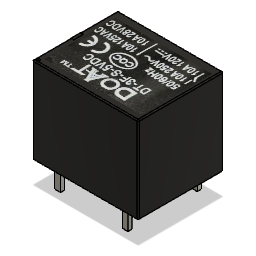
DOAT 5VOLT RELAY v1 (Autodesk Fusion 360 design; units mm, degrees)
Autodesk Fusion 360 part; units mm, degrees
sketch "Sketch1" plane through (0, 0, 0) normal (0, 1, 0) x (1, 0, 0)
  line L0 (9.375, -7.575) -> (-9.375, -7.575)
  line L1 (-9.375, -7.575) -> (-9.375, 7.575)
  line L2 (-9.375, 7.575) -> (9.375, 7.575)
  line L3 (9.375, 7.575) -> (9.375, -7.575)
  line L4 (9.375, -7.575) -> (-9.375, 7.575) construction
  line L5 (-9.375, -7.575) -> (9.375, 7.575) construction
  dimension "d1" = 15.15
  dimension "d2" = 18.75
  constraint horizontal L0
  constraint perpendicular L0 L1
  constraint parallel L0 L2
  constraint parallel L1 L3
  constraint coincident L4 origin
  constraint coincident L5 origin
  measures "d1" distance of L0.end L1.end
  measures "d2" distance of L1.end L2.end
extrude "Extrude1" add sketch "Sketch1" along normal blind 15.24
fillet "Fillet1" radius 0.2 4 edges at (9.375, 7.62, 7.575) (-9.375, 7.62, 7.575) (-9.375, 7.62, -7.575) (9.375, 7.62, -7.575) 1 faces at (3.125, 15.24, 2.525)
sketch "Sketch2" plane through (0, 0, 0) normal (0, -1, 0) x (1, 0, 0)
  arc A0 (-9.375, -7.375) -> (-9.175, -7.575) centre (-9.175, -7.375) ccw
  line L0 (-9.175, -7.575) -> (9.175, -7.575)
  arc A1 (9.175, -7.575) -> (9.375, -7.375) centre (9.175, -7.375) ccw
  line L1 (9.375, -7.375) -> (9.375, 7.375)
  arc A2 (9.375, 7.375) -> (9.175, 7.575) centre (9.175, 7.375) ccw
  line L2 (9.175, 7.575) -> (-9.175, 7.575)
  arc A3 (-9.175, 7.575) -> (-9.375, 7.375) centre (-9.175, 7.375) ccw
  line L3 (-9.375, 7.375) -> (-9.375, -7.375)
  line L4 (6.5, -6.5) -> (-6.5, -6.5) construction
  line L5 (-6.5, -6.5) -> (-6.5, 6.5) construction
  line L6 (-6.5, 6.5) -> (6.5, 6.5) construction
  line L7 (6.5, 6.5) -> (6.5, -6.5) construction
  line L8 (6.5, -6.5) -> (-6.5, 6.5) construction
  line L9 (-6.5, -6.5) -> (6.5, 6.5) construction
  line L10 (-6.5, 6.5) -> (-5.5, 6.5)
  line L11 (-5.5, 6.5) -> (-5.5, 5.8)
  line L12 (-5.5, 5.8) -> (-6.5, 5.8)
  line L13 (-6.5, 5.8) -> (-6.5, 6.5)
  line L14 (6.5, 5.8) -> (5.5, 5.8)
  line L15 (5.5, 6.5) -> (6.5, 6.5)
  line L16 (5.5, 5.8) -> (5.5, 6.5)
  line L17 (6.5, 6.5) -> (6.5, 5.8)
  line L18 (-5.5, -6.5) -> (-6.5, -6.5)
  line L19 (-6.5, -5.8) -> (-5.5, -5.8)
  line L20 (-6.5, -6.5) -> (-6.5, -5.8)
  line L21 (-5.5, -5.8) -> (-5.5, -6.5)
  line L22 (6.5, -6.5) -> (5.5, -6.5)
  line L23 (5.5, -5.8) -> (6.5, -5.8)
  line L24 (5.5, -6.5) -> (5.5, -5.8)
  line L25 (6.5, -5.8) -> (6.5, -6.5)
  dimension "d7" = 13
  dimension "d8" = 13
  dimension "d9" = 1
  dimension "d10" = 0.7
  dimension "d13" = 12
  dimension "d14" = -12.3
  constraint horizontal L4
  constraint perpendicular L4 L5
  constraint parallel L4 L6
  constraint parallel L5 L7
  constraint coincident L8 origin
  constraint coincident L9 origin
  constraint horizontal L10
  constraint vertical L11
  constraint horizontal L12
  constraint vertical L13
  measures "d7" distance of L5.end L6.end
  measures "d8" distance of L4.end L5.end
  measures "d9" distance of L5.end L10.end
  measures "d10" distance of L5.end L12.end
extrude "Extrude2" add sketch "Sketch2" along normal blind 4 contours L10 L11 L12 L13 | L14 L15 L16 L17 | L18 L19 L20 L21 | L22 L23 L24 L25
chamfer "Chamfer1" distance 0.2 angle 45 8 edges at (5.5, -4, 6.15) (6, -4, 6.5) (6.5, -4, 6.15) (6, -4, 5.8) (6, -4, -5.8) (6.5, -4, -6.15) (6, -4, -6.5) (5.5, -4, -6.15) 2 faces at (-6.1667, -4, 6.2667) (-5.8333, -4, -6.2667)
sketch "Sketch3" plane through (0, 0, 0) normal (0, -1, 0) x (1, 0, 0)
  line L0 (6.5, -5.8) -> (6.5, -6.5)
  line L1 (6.5, -6.5) -> (5.5, -6.5)
  line L2 (5.5, -6.5) -> (5.5, -5.8)
  line L3 (5.5, -5.8) -> (6.5, -5.8)
  line L4 (-6.5, 5.8) -> (-6.5, 6.5)
  line L5 (-6.5, 6.5) -> (-5.5, 6.5)
  line L6 (-5.5, 6.5) -> (-5.5, 5.8)
  line L7 (-5.5, 5.8) -> (-6.5, 5.8)
  line L8 (-5.5, -5.8) -> (-5.5, -6.5)
  line L9 (-5.5, -6.5) -> (-6.5, -6.5)
  line L10 (-6.5, -6.5) -> (-6.5, -5.8)
  line L11 (-6.5, -5.8) -> (-5.5, -5.8)
  line L12 (6.5, 6.5) -> (6.5, 5.8)
  line L13 (6.5, 5.8) -> (5.5, 5.8)
  line L14 (5.5, 5.8) -> (5.5, 6.5)
  line L15 (5.5, 6.5) -> (6.5, 6.5)
  arc A0 (-9.375, -7.375) -> (-9.175, -7.575) centre (-9.175, -7.375) ccw
  line L16 (-9.175, -7.575) -> (9.175, -7.575)
  arc A1 (9.175, -7.575) -> (9.375, -7.375) centre (9.175, -7.375) ccw
  line L17 (9.375, -7.375) -> (9.375, 7.375)
  arc A2 (9.375, 7.375) -> (9.175, 7.575) centre (9.175, 7.375) ccw
  line L18 (9.175, 7.575) -> (-9.175, 7.575)
  arc A3 (-9.175, 7.575) -> (-9.375, 7.375) centre (-9.175, 7.375) ccw
  line L19 (-9.375, 7.375) -> (-9.375, -7.375)
  line L20 (0, 0) -> (-9.375, 0) construction
  line L21 (-7.375, -0.5) -> (-8.075, -0.5)
  line L22 (-8.075, -0.5) -> (-8.075, 0.5)
  line L23 (-8.075, 0.5) -> (-7.375, 0.5)
  line L24 (-7.375, 0.5) -> (-7.375, -0.5)
  line L25 (-7.375, -0.5) -> (-8.075, 0.5) construction
  line L26 (-8.075, -0.5) -> (-7.375, 0.5) construction
  point P0 (-7.725, 0)
  dimension "d20" = 0.7
  dimension "d21" = 1
  constraint coincident L20.start origin
  constraint midpoint L19 L20.end
  constraint horizontal L21
  constraint perpendicular L21 L22
  constraint parallel L21 L23
  constraint parallel L22 L24
  constraint coincident L25 P0
  constraint coincident L26 P0
  measures "d20" distance of L22.end L23.end
  measures "d21" distance of L21.end L22.end
extrude "Extrude3" add sketch "Sketch3" along normal blind 4 contours L21 L22 L23 L24
chamfer "Chamfer2" distance 0.2 angle 45 4 edges at (-7.725, -4, -0.5) (-8.075, -4, 0) (-7.725, -4, 0.5) (-7.375, -4, 0)
sketch "Sketch4" plane through (0, 0, 0) normal (0, -1, 0) x (1, 0, 0)
  line L0 (-7.375, 0.5) -> (-7.375, -0.5)
  line L1 (-7.375, -0.5) -> (-8.075, -0.5)
  line L2 (-8.075, -0.5) -> (-8.075, 0.5)
  line L3 (-8.075, 0.5) -> (-7.375, 0.5)
  line L4 (6.5, -5.8) -> (6.5, -6.5)
  line L5 (6.5, -6.5) -> (5.5, -6.5)
  line L6 (5.5, -6.5) -> (5.5, -5.8)
  line L7 (5.5, -5.8) -> (6.5, -5.8)
  line L8 (-6.5, 5.8) -> (-6.5, 6.5)
  line L9 (-6.5, 6.5) -> (-5.5, 6.5)
  line L10 (-5.5, 6.5) -> (-5.5, 5.8)
  line L11 (-5.5, 5.8) -> (-6.5, 5.8)
  line L12 (-5.5, -5.8) -> (-5.5, -6.5)
  line L13 (-5.5, -6.5) -> (-6.5, -6.5)
  line L14 (-6.5, -6.5) -> (-6.5, -5.8)
  line L15 (-6.5, -5.8) -> (-5.5, -5.8)
  line L16 (6.5, 6.5) -> (6.5, 5.8)
  line L17 (6.5, 5.8) -> (5.5, 5.8)
  line L18 (5.5, 5.8) -> (5.5, 6.5)
  line L19 (5.5, 6.5) -> (6.5, 6.5)
  arc A0 (-9.375, -7.375) -> (-9.175, -7.575) centre (-9.175, -7.375) ccw
  line L20 (-9.175, -7.575) -> (9.175, -7.575)
  arc A1 (9.175, -7.575) -> (9.375, -7.375) centre (9.175, -7.375) ccw
  line L21 (9.375, -7.375) -> (9.375, 7.375)
  arc A2 (9.375, 7.375) -> (9.175, 7.575) centre (9.175, 7.375) ccw
  line L22 (9.175, 7.575) -> (-9.175, 7.575)
  arc A3 (-9.175, 7.575) -> (-9.375, 7.375) centre (-9.175, 7.375) ccw
  line L23 (-9.375, 7.375) -> (-9.375, -7.375)
  circle A4 centre (-6, 0) radius 0.75
  dimension "d25" = 1.5
  measures "d25" diameter of A4
extrude "Extrude4" cut sketch "Sketch4" against normal blind 0.1 contours A4
sketch "Sketch5" plane through (0, 0.1, 0) normal (0, -1, 0) x (1, 0, 0)
  circle A0 centre (-6, 0) radius 0.75
  circle A1 centre (-6, 0) radius 0.1
  constraint concentric A0 A1
extrude "Extrude5" add sketch "Sketch5" along normal blind 0.1 contours A1
sketch "Sketch6" plane through (0, 15.24, 0) normal (0, 1, 0) x (-1, 0, 0)
  line L0 (-9.175, -7.375) -> (9.175, -7.375)
  line L1 (9.175, -7.375) -> (9.175, 7.375)
  line L2 (9.175, 7.375) -> (-9.175, 7.375)
  line L3 (-9.175, 7.375) -> (-9.175, -7.375)
  line L4 (8.7536, 0.8698) -> (9.5964, 0.8698)
  line L5 (9.5964, 0.8698) -> (9.5964, -0.8698)
  line L6 (9.5964, -0.8698) -> (8.7536, -0.8698)
  line L7 (8.7536, -0.8698) -> (8.7536, 0.8698)
  line L8 (8.7536, 0.8698) -> (9.5964, -0.8698) construction
  line L9 (9.5964, 0.8698) -> (8.7536, -0.8698) construction
  circle A0 centre (8.8509, 7.0451) radius 0.2772
  point P0 (9.175, 0)
  constraint horizontal L4
  constraint perpendicular L4 L5
  constraint parallel L4 L6
  constraint parallel L5 L7
  constraint coincident L8 P0
  constraint coincident L9 P0
  constraint midpoint L1 P0
extrude "Extrude6" cut sketch "Sketch6" against normal blind 0.1 contours L1 L4 L6 L7 | L1 L4 L5 L6 | A0
